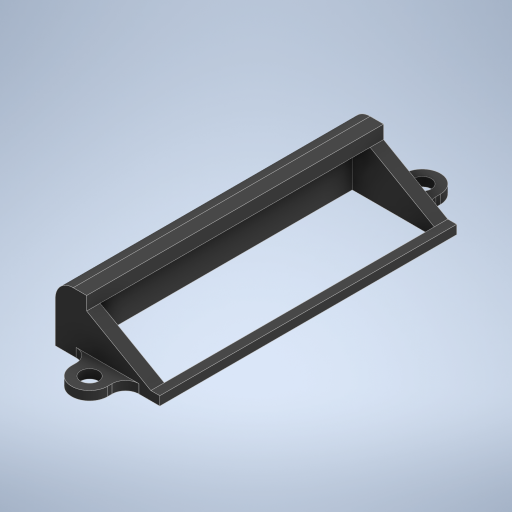
# Autodesk Inventor part: Clamp_Holder
Saved by Autodesk Inventor 2023 (Build 270158000, 158)
## iProperties
Created: 2024-07-31
Part Number: Clamp_Holder
Material: Generic
Document SubType Name: Modeling
Designer: Swoby
Density: 1 g/cm^3
Appearance: Default
Author: Swoby
Autodesk Inventor part; units mm, degrees
ref_plane "YZ Plane" through (0, 0, 0) normal (1, 0, 0) x (0, 1, 0)
ref_plane "XZ Plane" through (0, 0, 0) normal (0, 1, 0) x (-1, 0, 0)
ref_plane "XY Plane" through (0, 0, 0) normal (0, 0, 1) x (1, 0, 0)
sketch "Sketch1" plane through (0, 0, 0) normal (0, 0, 1) x (1, 0, 0)
  line L0 (0, 0) -> (-18.3, 0)
  line L1 (-18.3, 0) -> (-18.3, 7.2)
  line L2 (-15.3, 10.2) -> (-14.3, 10.2)
  line L3 (0, 10.2) -> (0, 2)
  arc A0 (-15.3, 10.2) -> (-18.3, 7.2) centre (-15.3, 7.2) ccw
  line L4 (-14.3, 10.2) -> (-14.3, 2)
  line L5 (-14.3, 2) -> (0, 2)
  line L6 (-14.3, 10.2) -> (0, 10.2)
  line L7 (0, 2) -> (0, 0)
  line L8 (-14.3, 10.2) -> (-14.3, 13.2)
  line L9 (-21.3, 0) -> (-21.3, 9.2)
  line L10 (-17.3, 13.2) -> (-14.3, 13.2)
  arc A1 (-17.3, 13.2) -> (-21.3, 9.2) centre (-17.3, 9.2) ccw
  line L11 (-21.3, 0) -> (-18.3, 0)
  line L12 (0, 0) -> (2, 0)
  line L13 (2, 0) -> (2, 2)
  line L14 (2, 2) -> (0, 2)
  line L15 (0, 2) -> (0, 0)
  dimension "d0" = 3
  dimension "d1" = 18.3
  dimension "d2" = 10.2
  dimension "d3" = 4
  dimension "d4" = 2
  dimension "d5" = 3
  dimension "d6" = 3
  dimension "d7" = 4
  dimension "d10" = 2
  dimension "d11" = 2
  constraints: 32 end point, 10 perpendicular, 5 tangent, 4 point on circle, 3 horizontal, 3 vertical, 2 centre point, 2 parallel
  measures "d0" radius of A0
  measures "d1" distance between parallel lines of L3 L1
  measures "d2" distance of L3.start L0.start
  measures "d3" distance between parallel lines of L1 L4
  measures "d4" distance between parallel lines of L0 L5
  measures "d5" distance of L2.end L8.end
  measures "d6" distance between parallel lines of L9 L1
  measures "d7" radius of A1
  measures "d10" distance of L14.end L13.end
  measures "d11" distance of L12.end L13.end
extrude "Extrusion1" add sketch "Sketch1" along normal blind 60.2 contours L7 L14 L13 L12 | L11 L9 A1 L10 L8 L2 A0 L1
sketch "Sketch2" plane through (0, 0, 60.2) normal (0, 0, 1) x (1, 0, 0)
  line L0 (-14.3, 10.2) -> (-14.3, 13.2) projected
  line L1 (-14.3, 13.2) -> (-17.3, 13.2) projected
  arc A0 (-17.3, 13.2) -> (-21.3, 9.2) centre (-17.3, 9.2) ccw projected
  line L2 (-21.3, 9.2) -> (-21.3, 0) projected
  line L3 (-21.3, 0) -> (-18.3, 0) projected
  line L4 (-18.3, 0) -> (-18.3, 7.2) projected
  arc A1 (-15.3, 10.2) -> (-18.3, 7.2) centre (-15.3, 7.2) ccw projected
  line L5 (-15.3, 10.2) -> (-14.3, 10.2) projected
  line L6 (0, 2) -> (0, 0) projected
  line L7 (0, 0) -> (2, 0) projected
  line L8 (2, 0) -> (2, 2) projected
  line L9 (2, 2) -> (0, 2) projected
  line L10 (0, 2) -> (-18.3, 2)
  line L11 (-18.3, 0) -> (0, 0)
  line L12 (-14.3, 10.2) -> (0, 2)
  constraints: 6 end point, 1 horizontal, 1 parallel, 1 point on line
extrude "Extrusion2" add sketch "Sketch2" along normal blind 3
sketch "Sketch3" plane through (0, 0, 0) normal (0, 0, -1) x (-1, 0, 0)
  line L0 (0, 2) -> (0, 0) projected
  line L1 (-2, 2) -> (0, 2) projected
  line L2 (-2, 0) -> (-2, 2) projected
  line L3 (0, 0) -> (-2, 0) projected
  line L4 (18.3, 0) -> (18.3, 7.2) projected
  line L5 (0, 2) -> (0, 0) projected
  line L6 (18.3, 0) -> (0, 0) projected
  line L7 (14.3, 10.2) -> (14.3, 13.2) projected
  line L8 (15.3, 10.2) -> (14.3, 10.2) projected
  arc A0 (18.3, 7.2) -> (15.3, 10.2) centre (15.3, 7.2) ccw projected
  line L9 (18.3, 0) -> (18.3, 7.2) projected
  line L10 (21.3, 0) -> (18.3, 0) projected
  line L11 (21.3, 9.2) -> (21.3, 0) projected
  arc A1 (21.3, 9.2) -> (17.3, 13.2) centre (17.3, 9.2) ccw projected
  line L12 (14.3, 13.2) -> (17.3, 13.2) projected
  line L13 (15.3, 10.2) -> (14.3, 10.2) projected
  line L14 (0, 2) -> (14.3, 10.2) projected
  arc A2 (18.3, 7.2) -> (15.3, 10.2) centre (15.3, 7.2) ccw projected
extrude "Extrusion3" add sketch "Sketch3" along normal blind 3
sketch "Sketch4" plane through (-21.3, 0, 63.2) normal (0, -1, 0) x (1, 0, 0)
  circle A0 centre (11.65, 4) radius 2
  line L0 (3, -63.2) -> (3, -3) projected
  line L1 (3, -3) -> (21.3, -3) projected
  line L2 (21.3, -63.2) -> (21.3, -3) projected
  line L3 (21.3, -63.2) -> (3, -63.2) projected
  line L4 (0, -66.2) -> (0, 0) projected
  line L5 (23.3, -66.2) -> (0, -66.2) projected
  line L6 (23.3, -66.2) -> (23.3, 0) projected
  line L7 (0, 0) -> (23.3, 0) projected
  line L8 (11.65, 0) -> (11.65, 4) construction
  arc A1 (11.65, 0) -> (15.65, 4) centre (11.65, 4) ccw construction
  line L9 (7.65, 4) -> (7.65, 0)
  line L10 (15.65, 4) -> (15.65, 0)
  arc A2 (7.65, 4) -> (11.65, 0) centre (11.65, 4) ccw construction
  arc A3 (15.65, 4) -> (7.65, 4) centre (11.65, 4) ccw
  dimension "d16" = 4
  dimension "d17" = 4
  constraints: 6 end point, 6 point on circle, 4 centre point, 4 tangent, 2 coincident, 2 perpendicular, 2 point on line, 1 midpoint, 1 vertical
  measures "d16" diameter of A0
  measures "d17" distance of L8.start L8.end
extrude "Extrusion4" add sketch "Sketch4" against normal up to surface (2 mm away) contours L9 A3 L10 L7
ref_plane "Work Plane1" through (0, 0, 30.1) normal (0, 0, -1) x (-1, 0, 0)
mirror "Mirror1" about plane through (0, 0, 30.1) normal (0, 0, -1) of "Extrusion4"
fillet "Fillet1" radius 3 4 edges at (-13.65, 1, -3) (-5.65, 1, -3) (-5.65, 1, 63.2) (-13.65, 1, 63.2)
body "Solid1"
